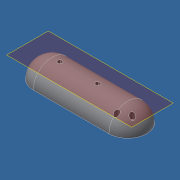
# Autodesk Inventor part: P1704_005_mainGaucheExterieur
Saved by Autodesk Inventor 2019 (Build 230136000, 136)
## iProperties
Created: 2019-05-02
Part Number: P1704_005_mainGaucheExterieur
Project: Nom Projet
Material: .
Description: Nom pièce
Document SubType Name: Modeling
Designer: Joan.MAILLARD
Authority: brut Ø
Density: 0.001 g/cm^3
Appearance: Par défaut
Material number: ---
Author: Joan.MAILLARD
Autodesk Inventor part; units mm, degrees
ref_plane "Plan YZ" through (0, 0, 0) normal (1, 0, 0) x (0, 1, 0)
ref_plane "Plan XZ" through (0, 0, 0) normal (0, 1, 0) x (-1, 0, 0)
ref_plane "Plan XY" through (0, 0, 0) normal (0, 0, 1) x (1, 0, 0)
sketch "Esquisse1" plane through (0, 0, 0) normal (0, 0, 1) x (1, 0, 0)
  arc A0 (25, 25) -> (0, 0) centre (25, 0) ccw
  line L0 (25, 25) -> (125, 25)
  arc A1 (150, 0) -> (125, 25) centre (125, 0) ccw
  line L1 (0, 0) -> (150, 0)
  dimension "d0" = 100
  dimension "d1" = 25
  constraints: 5 point on circle, 4 end point, 2 centre point, 2 horizontal, 2 point on line, 2 tangent
  measures "d0" distance of L0.start L0.end
  measures "d1" distance from line of L1.start L0
revolve "Révolution1" add sketch "Esquisse1" angle 180 about axis through (0, 0, 0) along (1, 0, 0)
ref_plane "Plan de construction1" through (125, 25, 25) normal (0, 0, -1) x (-1, 0, 0)
sketch "Esquisse6" plane through (125, 25, 25) normal (0, 0, -1) x (-1, 0, 0)
  line L0 (86.7668, -25) -> (88.3834, -22.2)
  line L1 (88.3834, -22.2) -> (91.6166, -22.2)
  line L2 (91.6166, -22.2) -> (93.2332, -25)
  line L3 (93.2332, -25) -> (91.6166, -27.8)
  line L4 (91.6166, -27.8) -> (88.3834, -27.8)
  line L5 (88.3834, -27.8) -> (86.7668, -25)
  line L6 (100, 0) -> (100, -50) projected
  line L7 (36.7668, -25) -> (38.3834, -22.2)
  line L8 (38.3834, -22.2) -> (41.6166, -22.2)
  line L9 (41.6166, -22.2) -> (43.2332, -25)
  line L10 (43.2332, -25) -> (41.6166, -27.8)
  line L11 (41.6166, -27.8) -> (38.3834, -27.8)
  line L12 (38.3834, -27.8) -> (36.7668, -25)
  line L13 (40, -25) -> (36.7668, -25) construction
  line L14 (100, -25) -> (19.1163, -25) construction
  line L15 (90, -25) -> (86.7668, -25) construction
  point P0 (125, -25)
  dimension "d4" = 5.6
  dimension "d5" = 10
  dimension "d6" = 50
  dimension "d7" = 5.6
  constraints: 30 end point, 2 horizontal, 2 point on line, 1 collinear, 1 midpoint, 26 other
  measures "d4" distance between parallel lines of L3 L0
  measures "d5" distance from line of L6 L15.start
  measures "d6" distance of L13.start L15.start
  measures "d7" distance between parallel lines of L10 L7
extrude "Extrusion1" cut sketch "Esquisse6" along normal blind 12
sketch "Esquisse7" plane through (125, 25, 25) normal (0, 0, -1) x (-1, 0, 0)
  circle A0 centre (90, -25) radius 3.2332 construction
  circle A1 centre (40, -25) radius 3.2332 construction
  circle A2 centre (90, -25) radius 1.7
  circle A3 centre (40, -25) radius 1.7
  point P0 (125, -25)
  point P1 (88.3834, -22.2)
  point P2 (38.3834, -22.2)
  point P3 (41.6166, -27.8)
  point P4 (38.3834, -27.8)
  point P5 (91.6166, -27.8)
  point P6 (88.3834, -27.8)
  dimension "d10" = 3.4
  dimension "d11" = 3.4
  constraints: 6 point on circle, 4 centre point, 2 coincident
  measures "d10" diameter of A2
  measures "d11" diameter of A3
extrude "Extrusion2" cut sketch "Esquisse7" along normal blind 25
sketch "Esquisse8" plane through (125, 25, 25) normal (0, 0, -1) x (-1, 0, 0)
  line L0 (-0.0645, -24.9628) -> (-43.3013, 0) construction
  line L1 (-43.3013, 0) -> (-55.8013, -21.6506) construction
  line L2 (-55.8013, -21.6506) -> (9.1506, -59.1506) construction
  line L3 (9.1506, -59.1506) -> (21.6506, -37.5) construction
  line L4 (21.6506, -37.5) -> (-0.0645, -24.9628) construction
  arc A0 (0, 0) -> (0, -50) centre (0, -25) ccw projected
  line L5 (0, 0) -> (0, -50) projected
  line L6 (100, 0) -> (0, 0) projected
  line L7 (-13.9282, -33.1244) -> (-0.9378, -40.6244) construction
  circle A1 centre (-13.9282, -33.1244) radius 1.7
  circle A2 centre (-0.9378, -40.6244) radius 1.7
  point P0 (125, -25)
  dimension "d14" = 300
  dimension "d15" = 14
  dimension "d16" = 18
  dimension "d17" = 33
  dimension "d18" = 3.4
  dimension "d19" = 3.4
  constraints: 12 end point, 4 perpendicular, 3 point on line, 2 centre point, 2 coincident, 1 midpoint, 1 parallel, 1 point on circle, 1 tangent
  measures "d15" distance between parallel lines of L0 L7
  measures "d16" distance from line of L7.end L3
  measures "d17" distance from line of L7.start L3
  measures "d18" diameter of A1
  measures "d19" diameter of A2
extrude "Extrusion3" cut sketch "Esquisse8" along normal blind 25 contours A2 L5 | L5 A2 | A1
sketch "Esquisse9" plane through (125, 25, 25) normal (0, 0, -1) x (-1, 0, 0)
  circle A0 centre (-13.9282, -33.1244) radius 3.25
  circle A1 centre (-0.9378, -40.6244) radius 3.25
  circle A2 centre (-13.9282, -33.1244) radius 1.7 projected
  circle A3 centre (-0.9378, -40.6244) radius 1.7 projected
  point P0 (125, -25)
  dimension "d22" = 6.5
  dimension "d23" = 6.5
  constraints: 2 centre point, 2 concentric
  measures "d22" diameter of A0
  measures "d23" diameter of A1
extrude "Extrusion4" cut sketch "Esquisse9" along normal blind 12.5
equation "\"d7\" = d4"
equation "\"d11\" = d10"
equation "\"d19\" = d18"
equation "\"d23\" = d22"
